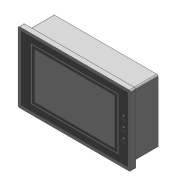
# Autodesk Inventor part: IHM SANKOON 4 POL
Saved by Autodesk Inventor 2022 (Build 260153000, 153)
## iProperties
Created: 2022-08-06
Part Number: IHM SANKOON 4 POL
Material: Genérico
Document SubType Name: Modeling
Designer: Tiago
Density: 1 g/cm^3
Appearance: Padrão
Author: Tiago
Autodesk Inventor part; units mm, degrees
ref_plane "YZ Plane" through (0, 0, 0) normal (1, 0, 0) x (0, 1, 0)
ref_plane "XZ Plane" through (0, 0, 0) normal (0, 1, 0) x (-1, 0, 0)
ref_plane "XY Plane" through (0, 0, 0) normal (0, 0, 1) x (1, 0, 0)
sketch "Esboço8" plane through (0, 0, 0) normal (0, 0, 1) x (1, 0, 0)
  line L0 (-64.5, 38.65) -> (64.5, 38.65)
  line L1 (64.5, 38.65) -> (64.5, -38.65)
  line L2 (64.5, -38.65) -> (-64.5, -38.65)
  line L3 (-64.5, -38.65) -> (-64.5, 38.65)
  line L4 (-64.5, 38.65) -> (64.5, -38.65) construction
  line L5 (64.5, 38.65) -> (-64.5, -38.65) construction
  point P0 (0, 0)
  dimension "d24" = 129
  dimension "d25" = 77.3
  constraints: 12 end point, 2 midpoint, 2 parallel, 1 horizontal, 1 perpendicular
  measures "d24" distance of L0.start L0.end
  measures "d25" distance of L2.end L0.start
extrude "Extrusão6" add sketch "Esboço8" along normal blind 38
sketch "Esboço9" plane through (0, 0, 38) normal (0, 0, 1) x (1, 0, 0)
  line L0 (-69, 43) -> (69, 43)
  line L1 (69, 43) -> (69, -43)
  line L2 (69, -43) -> (-69, -43)
  line L3 (-69, -43) -> (-69, 43)
  line L4 (-69, 43) -> (69, -43) construction
  line L5 (69, 43) -> (-69, -43) construction
  point P0 (0, 0)
  dimension "d28" = 138
  dimension "d29" = 86
  constraints: 12 end point, 2 midpoint, 2 parallel, 1 horizontal, 1 perpendicular
  measures "d28" distance of L0.start L0.end
  measures "d29" distance of L2.end L0.start
extrude "Extrusão7" add sketch "Esboço9" against normal blind 6
sketch "Esboço10" plane through (0, 0, 38) normal (0, 0, 1) x (1, 0, 0)
  line L0 (-65.5, 39.5) -> (65.5, 39.5)
  line L1 (65.5, 39.5) -> (65.5, -39.5)
  line L2 (65.5, -39.5) -> (-65.5, -39.5)
  line L3 (-65.5, -39.5) -> (-65.5, 39.5)
  line L4 (-65.5, 39.5) -> (65.5, -39.5) construction
  line L5 (65.5, 39.5) -> (-65.5, -39.5) construction
  line L6 (-69, 43) -> (-69, -43) projected
  line L7 (69, 43) -> (-69, 43) projected
  point P0 (0, 0)
  dimension "d32" = 3.5
  dimension "d33" = 3.5
  constraints: 12 end point, 2 midpoint, 2 parallel, 1 horizontal, 1 perpendicular
  measures "d32" distance between parallel lines of L6 L3
  measures "d33" distance between parallel lines of L7 L0
extrude "Extrusão8" cut sketch "Esboço10" against normal blind 0.25
fillet "Arredondamento1" radius 2 4 edges at (69, 43, 35) (-69, 43, 35) (-69, -43, 35) (69, -43, 35)
sketch "Esboço11" plane through (0, 0, 37.75) normal (0, 0, 1) x (1, 0, 0)
  line L0 (-49, 28) -> (49, 28)
  line L1 (49, 28) -> (49, -28)
  line L2 (49, -28) -> (-49, -28)
  line L3 (-49, -28) -> (-49, 28)
  line L4 (-49, 28) -> (49, -28) construction
  line L5 (49, 28) -> (-49, -28) construction
  line L6 (67, 43) -> (-67, 43) projected
  line L7 (69, -41) -> (69, 41) projected
  point P0 (0, 0)
  dimension "d38" = 15
  dimension "d39" = 20
  constraints: 12 end point, 2 midpoint, 2 parallel, 1 horizontal, 1 perpendicular
  measures "d38" distance between parallel lines of L6 L0
  measures "d39" distance between parallel lines of L7 L1
extrude "Extrusão9" cut sketch "Esboço11" against normal blind 0.01
sketch "Esboço12" plane through (0, 0, 37.75) normal (0, 0, 1) x (1, 0, 0)
  line L0 (-52.5, -31) -> (52.5, -31)
  line L1 (52.5, -31) -> (52.5, 31)
  line L2 (52.5, 31) -> (-52.5, 31)
  line L3 (-52.5, 31) -> (-52.5, -31)
  line L4 (-52.5, -31) -> (52.5, 31) construction
  line L5 (52.5, -31) -> (-52.5, 31) construction
  line L6 (-53.5, 32) -> (53.5, 32)
  line L7 (53.5, 32) -> (53.5, -32)
  line L8 (53.5, -32) -> (-53.5, -32)
  line L9 (-53.5, -32) -> (-53.5, 32)
  point P0 (0, 0)
  dimension "d42" = 105
  dimension "d43" = 62
  dimension "d44" = 1
  constraints: 20 end point, 4 parallel, 2 midpoint, 2 perpendicular, 1 horizontal, 3 other
  measures "d42" distance of L1.end L2.end
  measures "d43" distance of L2.end L0.start
  measures "d44" distance between parallel lines of L2 L6
extrude "Extrusão10" add sketch "Esboço12" along normal blind 0.01
sketch "Esboço13" plane through (0, 0, 37.75) normal (0, 0, 1) x (1, 0, 0)
  line L0 (-53.5, 32) -> (53.5, 32) projected
  circle A0 centre (59.75, 12) radius 1.25
  circle A1 centre (59.75, 0) radius 1.25
  circle A2 centre (59.75, -12) radius 1.25
  point P0 (0, 0)
  dimension "d47" = 2.5
  dimension "d48" = 2.5
  dimension "d49" = 2.5
  constraints: 3 centre point
  measures "d47" diameter of A0
  measures "d48" diameter of A1
  measures "d49" diameter of A2
extrude "Extrusão11" add sketch "Esboço13" along normal blind 0.01
sketch "Esboço14" plane through (0, 0, 37.75) normal (0, 0, 1) x (1, 0, 0)
  line L0 (56.368, 8.4925) -> (65.06, 8.4925) construction
  line L1 (65.06, 8.4925) -> (65.06, 5.4445) construction
  line L2 (65.06, 5.4445) -> (56.368, 5.4445) construction
  line L3 (56.368, 5.4445) -> (56.368, 8.4925) construction
  line L4 (56.2897, -3.4254) -> (64.9816, -3.4254) construction
  line L5 (64.9816, -3.4254) -> (64.9816, -6.4734) construction
  line L6 (64.9816, -6.4734) -> (56.2897, -6.4734) construction
  line L7 (56.2897, -6.4734) -> (56.2897, -3.4254) construction
  line L8 (56.4183, -18.2349) -> (56.4183, -15.1869) construction
  line L9 (56.4183, -15.1869) -> (65.1102, -15.1869) construction
  line L10 (65.1102, -15.1869) -> (65.1102, -18.2349) construction
  line L11 (65.1102, -18.2349) -> (56.4183, -18.2349) construction
  line L12 (56.5829, 6.4925) -> (56.5829, 8.4925)
  line L13 (56.5829, 8.4925) -> (57.3375, 8.4925)
  spline S0 degree 2 poles (57.3375, 8.4925) (57.5372, 8.4925) (57.6424, 8.4727) knots 0 0 0 1 1 1
  spline S1 degree 2 poles (57.6424, 8.4727) (57.7902, 8.4483) (57.9884, 8.3111) (58.1104, 8.0626) (58.1104, 7.9132) knots 0 0 0 1 2 3 3 3
  spline S2 degree 2 poles (58.1104, 7.9132) (58.1104, 7.6586) (57.7857, 7.305) (57.3619, 7.305) knots 0 0 0 1 2 2 2
  line L14 (57.3619, 7.305) -> (56.8482, 7.305)
  line L15 (56.8482, 7.305) -> (56.8482, 6.4925)
  line L16 (56.8482, 6.4925) -> (56.5829, 6.4925)
  line L17 (56.8482, 7.5413) -> (57.3649, 7.5413)
  spline S3 degree 2 poles (57.3649, 7.5413) (57.6226, 7.5413) (57.8375, 7.7318) (57.8375, 7.9056) knots 0 0 0 1 2 2 2
  spline S4 degree 2 poles (57.8375, 7.9056) (57.8375, 8.0306) (57.711, 8.2105) (57.6073, 8.2379) knots 0 0 0 1 2 2 2
  spline S5 degree 2 poles (57.6073, 8.2379) (57.5402, 8.2562) (57.3604, 8.2562) knots 0 0 0 1 1 1
  line L18 (57.3604, 8.2562) -> (56.8482, 8.2562)
  line L19 (56.8482, 8.2562) -> (56.8482, 7.5413)
  line L20 (58.7963, 6.4925) -> (58.2659, 8.4925)
  line L21 (58.2659, 8.4925) -> (58.5372, 8.4925)
  line L22 (58.5372, 8.4925) -> (58.8421, 7.1815)
  spline S6 degree 2 poles (58.8421, 7.1815) (58.8909, 6.9757) (58.9274, 6.7714) knots 0 0 0 1 1 1
  spline S7 degree 2 poles (58.9274, 6.7714) (59.0037, 7.0931) (59.0174, 7.1419) knots 0 0 0 1 1 1
  line L23 (59.0174, 7.1419) -> (59.397, 8.4925)
  line L24 (59.397, 8.4925) -> (59.7171, 8.4925)
  line L25 (59.7171, 8.4925) -> (60.0037, 7.4803)
  spline S8 degree 2 poles (60.0037, 7.4803) (60.1088, 7.1038) (60.1591, 6.7714) knots 0 0 0 1 1 1
  spline S9 degree 2 poles (60.1591, 6.7714) (60.1973, 6.962) (60.2582, 7.2074) knots 0 0 0 1 1 1
  line L26 (60.2582, 7.2074) -> (60.5707, 8.4925)
  line L27 (60.5707, 8.4925) -> (60.8375, 8.4925)
  line L28 (60.8375, 8.4925) -> (60.2918, 6.4925)
  line L29 (60.2918, 6.4925) -> (60.0326, 6.4925)
  line L30 (60.0326, 6.4925) -> (59.6149, 8.0169)
  spline S10 degree 2 poles (59.6149, 8.0169) (59.5601, 8.2074) (59.5509, 8.2516) knots 0 0 0 1 1 1
  spline S11 degree 2 poles (59.5509, 8.2516) (59.5174, 8.1144) (59.4915, 8.0169) knots 0 0 0 1 1 1
  line L31 (59.4915, 8.0169) -> (59.0692, 6.4925)
  line L32 (59.0692, 6.4925) -> (58.7963, 6.4925)
  line L33 (61.089, 6.4925) -> (61.089, 8.4925)
  line L34 (61.089, 8.4925) -> (61.9762, 8.4925)
  spline S12 degree 2 poles (61.9762, 8.4925) (62.243, 8.4925) (62.522, 8.3842) (62.6881, 8.1114) (62.6881, 7.9467) knots 0 0 0 1 2 3 3 3
  spline S13 degree 2 poles (62.6881, 7.9467) (62.6881, 7.7333) (62.4122, 7.4422) (62.1256, 7.4025) knots 0 0 0 1 2 2 2
  spline S14 degree 2 poles (62.1256, 7.4025) (62.2293, 7.3522) (62.2841, 7.3035) knots 0 0 0 1 1 1
  spline S15 degree 2 poles (62.2841, 7.3035) (62.4, 7.1967) (62.5037, 7.0367) knots 0 0 0 1 1 1
  line L35 (62.5037, 7.0367) -> (62.8497, 6.4925)
  line L36 (62.8497, 6.4925) -> (62.5189, 6.4925)
  line L37 (62.5189, 6.4925) -> (62.2537, 6.9086)
  spline S16 degree 2 poles (62.2537, 6.9086) (62.1378, 7.0885) (61.9884, 7.2791) (61.8695, 7.3568) (61.8085, 7.372) knots 0 0 0 1 2 3 3 3
  spline S17 degree 2 poles (61.8085, 7.372) (61.7628, 7.3812) (61.6607, 7.3812) knots 0 0 0 1 1 1
  line L38 (61.6607, 7.3812) -> (61.3543, 7.3812)
  line L39 (61.3543, 7.3812) -> (61.3543, 6.4925)
  line L40 (61.3543, 6.4925) -> (61.089, 6.4925)
  line L41 (61.3543, 7.6099) -> (61.9229, 7.6099)
  spline S18 degree 2 poles (61.9229, 7.6099) (62.1043, 7.6099) (62.3085, 7.6845) (62.4152, 7.8507) (62.4152, 7.9467) knots 0 0 0 1 2 3 3 3
  spline S19 degree 2 poles (62.4152, 7.9467) (62.4152, 8.0885) (62.2095, 8.2714) (61.9869, 8.2714) knots 0 0 0 1 2 2 2
  line L42 (61.9869, 8.2714) -> (61.3543, 8.2714)
  line L43 (61.3543, 8.2714) -> (61.3543, 7.6099)
  line L44 (56.5092, -5.4254) -> (56.5092, -3.4254)
  line L45 (56.5092, -3.4254) -> (57.3964, -3.4254)
  spline S20 degree 2 poles (57.3964, -3.4254) (57.6631, -3.4254) (57.9421, -3.5336) (58.1082, -3.8065) (58.1082, -3.9711) knots 0 0 0 1 2 3 3 3
  spline S21 degree 2 poles (58.1082, -3.9711) (58.1082, -4.1846) (57.8323, -4.4757) (57.5457, -4.5154) knots 0 0 0 1 2 2 2
  spline S22 degree 2 poles (57.5457, -4.5154) (57.6494, -4.5657) (57.7043, -4.6144) knots 0 0 0 1 1 1
  spline S23 degree 2 poles (57.7043, -4.6144) (57.8201, -4.7211) (57.9238, -4.8812) knots 0 0 0 1 1 1
  line L46 (57.9238, -4.8812) -> (58.2698, -5.4254)
  line L47 (58.2698, -5.4254) -> (57.939, -5.4254)
  line L48 (57.939, -5.4254) -> (57.6738, -5.0093)
  spline S24 degree 2 poles (57.6738, -5.0093) (57.5579, -4.8294) (57.4086, -4.6388) (57.2897, -4.5611) (57.2287, -4.5458) knots 0 0 0 1 2 3 3 3
  spline S25 degree 2 poles (57.2287, -4.5458) (57.1829, -4.5367) (57.0808, -4.5367) knots 0 0 0 1 1 1
  line L49 (57.0808, -4.5367) -> (56.7744, -4.5367)
  line L50 (56.7744, -4.5367) -> (56.7744, -5.4254)
  line L51 (56.7744, -5.4254) -> (56.5092, -5.4254)
  line L52 (56.7744, -4.308) -> (57.343, -4.308)
  spline S26 degree 2 poles (57.343, -4.308) (57.5244, -4.308) (57.7287, -4.2333) (57.8354, -4.0672) (57.8354, -3.9711) knots 0 0 0 1 2 3 3 3
  spline S27 degree 2 poles (57.8354, -3.9711) (57.8354, -3.8294) (57.6296, -3.6465) (57.407, -3.6465) knots 0 0 0 1 2 2 2
  line L53 (57.407, -3.6465) -> (56.7744, -3.6465)
  line L54 (56.7744, -3.6465) -> (56.7744, -4.308)
  line L55 (59.8354, -3.4254) -> (60.1006, -3.4254)
  line L56 (60.1006, -3.4254) -> (60.1006, -4.5809)
  spline S28 degree 2 poles (60.1006, -4.5809) (60.1006, -4.8827) (59.965, -5.2364) (59.6082, -5.459) (59.3186, -5.459) knots 0 0 0 1 2 3 3 3
  spline S29 degree 2 poles (59.3186, -5.459) (59.0381, -5.459) (58.6799, -5.2654) (58.5275, -4.898) (58.5275, -4.5809) knots 0 0 0 1 2 3 3 3
  line L57 (58.5275, -4.5809) -> (58.5275, -3.4254)
  line L58 (58.5275, -3.4254) -> (58.7927, -3.4254)
  line L59 (58.7927, -3.4254) -> (58.7927, -4.5794)
  spline S30 degree 2 poles (58.7927, -4.5794) (58.7927, -4.8385) (58.8887, -5.0855) (59.125, -5.2196) (59.2957, -5.2196) knots 0 0 0 1 2 3 3 3
  spline S31 degree 2 poles (59.2957, -5.2196) (59.5869, -5.2196) (59.8354, -4.9544) (59.8354, -4.5794) knots 0 0 0 1 2 2 2
  line L60 (59.8354, -4.5794) -> (59.8354, -3.4254)
  line L61 (60.5397, -5.4254) -> (60.5397, -3.4254)
  line L62 (60.5397, -3.4254) -> (60.811, -3.4254)
  line L63 (60.811, -3.4254) -> (61.8628, -4.9955)
  line L64 (61.8628, -4.9955) -> (61.8628, -3.4254)
  line L65 (61.8628, -3.4254) -> (62.1159, -3.4254)
  line L66 (62.1159, -3.4254) -> (62.1159, -5.4254)
  line L67 (62.1159, -5.4254) -> (61.8445, -5.4254)
  line L68 (61.8445, -5.4254) -> (60.7927, -3.8553)
  line L69 (60.7927, -3.8553) -> (60.7927, -5.4254)
  line L70 (60.7927, -5.4254) -> (60.5397, -5.4254)
  line L71 (58.06, -16.5192) -> (58.3253, -16.5863)
  spline S32 degree 2 poles (58.3253, -16.5863) (58.2414, -16.9125) (57.81, -17.2555) (57.4975, -17.2555) knots 0 0 0 1 2 2 2
  spline S33 degree 2 poles (57.4975, -17.2555) (57.1744, -17.2555) (56.7689, -16.9918) (56.557, -16.4933) (56.557, -16.2067) knots 0 0 0 1 2 3 3 3
  spline S34 degree 2 poles (56.557, -16.2067) (56.557, -15.8942) (56.7963, -15.4277) (57.2369, -15.1869) (57.5021, -15.1869) knots 0 0 0 1 2 3 3 3
  spline S35 degree 2 poles (57.5021, -15.1869) (57.8024, -15.1869) (58.2109, -15.4933) (58.2917, -15.7692) knots 0 0 0 1 2 2 2
  line L72 (58.2917, -15.7692) -> (58.0311, -15.8317)
  spline S36 degree 2 poles (58.0311, -15.8317) (57.9609, -15.6137) (57.6972, -15.414) (57.496, -15.414) knots 0 0 0 1 2 2 2
  spline S37 degree 2 poles (57.496, -15.414) (57.2658, -15.414) (56.9548, -15.635) (56.8298, -16.007) (56.8298, -16.2052) knots 0 0 0 1 2 3 3 3
  spline S38 degree 2 poles (56.8298, -16.2052) (56.8298, -16.4597) (56.9792, -16.8408) (57.2917, -17.0283) (57.4747, -17.0283) knots 0 0 0 1 2 3 3 3
  spline S39 degree 2 poles (57.4747, -17.0283) (57.6972, -17.0283) (58.0052, -16.7722) (58.06, -16.5192) knots 0 0 0 1 2 2 2
  spline S40 degree 2 poles (58.5722, -16.2479) (58.5722, -15.7494) (59.1073, -15.1869) (59.5295, -15.1869) knots 0 0 0 1 2 2 2
  spline S41 degree 2 poles (59.5295, -15.1869) (59.807, -15.1869) (60.2521, -15.4521) (60.4853, -15.9247) (60.4853, -16.225) knots 0 0 0 1 2 3 3 3
  spline S42 degree 2 poles (60.4853, -16.225) (60.4853, -16.5283) (60.2399, -17.0085) (59.7887, -17.2555) (59.5295, -17.2555) knots 0 0 0 1 2 3 3 3
  spline S43 degree 2 poles (59.5295, -17.2555) (59.246, -17.2555) (58.8009, -16.9826) (58.5722, -16.5116) (58.5722, -16.2479) knots 0 0 0 1 2 3 3 3
  spline S44 degree 2 poles (58.8451, -16.2509) (58.8451, -16.6122) (59.2338, -17.0283) (59.528, -17.0283) knots 0 0 0 1 2 2 2
  spline S45 degree 2 poles (59.528, -17.0283) (59.8268, -17.0283) (60.2125, -16.6091) (60.2125, -16.2219) knots 0 0 0 1 2 2 2
  spline S46 degree 2 poles (60.2125, -16.2219) (60.2125, -15.978) (60.0478, -15.6137) (59.7292, -15.414) (59.5311, -15.414) knots 0 0 0 1 2 3 3 3
  spline S47 degree 2 poles (59.5311, -15.414) (59.2506, -15.414) (58.8451, -15.7997) (58.8451, -16.2509) knots 0 0 0 1 2 2 2
  line L73 (60.8177, -17.2219) -> (60.8177, -15.2219)
  line L74 (60.8177, -15.2219) -> (61.2155, -15.2219)
  line L75 (61.2155, -15.2219) -> (61.6896, -16.6381)
  spline S48 degree 2 poles (61.6896, -16.6381) (61.7552, -16.8363) (61.7856, -16.9338) knots 0 0 0 1 1 1
  spline S49 degree 2 poles (61.7856, -16.9338) (61.8192, -16.8256) (61.8923, -16.6137) knots 0 0 0 1 1 1
  line L76 (61.8923, -16.6137) -> (62.3725, -15.2219)
  line L77 (62.3725, -15.2219) -> (62.7277, -15.2219)
  line L78 (62.7277, -15.2219) -> (62.7277, -17.2219)
  line L79 (62.7277, -17.2219) -> (62.4731, -17.2219)
  line L80 (62.4731, -17.2219) -> (62.4731, -15.5482)
  line L81 (62.4731, -15.5482) -> (61.8893, -17.2219)
  line L82 (61.8893, -17.2219) -> (61.6515, -17.2219)
  line L83 (61.6515, -17.2219) -> (61.0722, -15.5192)
  line L84 (61.0722, -15.5192) -> (61.0722, -17.2219)
  line L85 (61.0722, -17.2219) -> (60.8177, -17.2219)
  point P0 (0, 0)
  constraints: 6 other
extrude "Extrusão12" add sketch "Esboço14" along normal blind 0.01
fillet "Arredondamento2" radius 2 4 edges at (64.5, 38.65, 16) (-64.5, 38.65, 16) (64.5, -38.65, 16) (-64.5, -38.65, 16)
